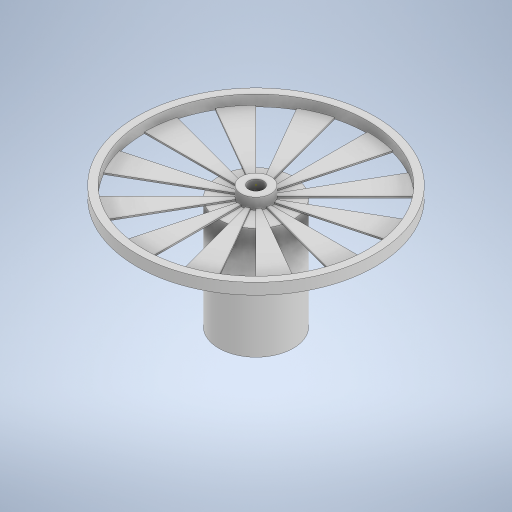
# Autodesk Inventor part: fan_num3
Saved by Autodesk Inventor 2024 (Build 280153000, 153)
## iProperties
Created: 2024-08-06
Part Number: fan_num3
Material: 일반
Document SubType Name: Modeling
Designer: chlqj
Density: 1 g/cm^3
Appearance: 기본값
Author: chlqj
Autodesk Inventor part; units mm, degrees
ref_plane "YZ Plane" through (0, 0, 0) normal (1, 0, 0) x (0, 1, 0)
ref_plane "XZ Plane" through (0, 0, 0) normal (0, 1, 0) x (-1, 0, 0)
ref_plane "XY Plane" through (0, 0, 0) normal (0, 0, 1) x (1, 0, 0)
sketch "스케치1" plane through (0, 0, 0) normal (0, 1, 0) x (-1, 0, 0)
  circle A0 centre (0, 0) radius 5
  dimension "d0" = 10
  constraints: 1 centre point, 1 coincident
  measures "d0" diameter of A0
extrude "돌출1" add sketch "스케치1" along normal blind 15
sketch "스케치2" plane through (0, 15, 0) normal (0, 1, 0) x (1, 0, 0)
  circle A0 centre (0, 0) radius 15
  circle A1 centre (0, 0) radius 16
  dimension "d3" = 30
  dimension "d4" = 32
  constraints: 2 centre point, 2 coincident
  measures "d3" diameter of A0
  measures "d4" diameter of A1
extrude "돌출2" add sketch "스케치2" along normal blind 1.5
sketch "스케치3" plane through (0, 15, 0) normal (0, 1, 0) x (1, 0, 0)
  line L0 (0, 0) -> (15, 0)
  circle A0 centre (0, 0) radius 15 projected
  line L1 (0, 0) -> (14.4889, 3.8823)
  line L2 (0, 0) -> (15, 0) construction
  line L3 (0, 0) -> (12.9904, 7.5)
  line L4 (0, 0) -> (15, 0) construction
  line L5 (0, 0) -> (10.6066, 10.6066)
  line L6 (0, 0) -> (15, 0) construction
  line L7 (0, 0) -> (7.5, 12.9904)
  line L8 (0, 0) -> (15, 0) construction
  line L9 (0, 0) -> (3.8823, 14.4889)
  line L10 (0, 0) -> (15, 0) construction
  line L11 (0, 0) -> (0, 15)
  line L12 (0, 0) -> (-3.8823, 14.4889)
  line L13 (0, 0) -> (-7.5, 12.9904)
  line L14 (0, 0) -> (-10.6066, 10.6066)
  line L15 (0, 0) -> (-12.9904, 7.5)
  line L16 (0, 0) -> (-14.2878, 3.8284)
  line L17 (0, 0) -> (-12.9904, -7.5)
  line L18 (0, 0) -> (-7.5, -12.9904)
  line L19 (0, 0) -> (0, -15)
  line L20 (0, 0) -> (10.6066, -10.6066)
  line L21 (0, 0) -> (12.9904, -7.5)
  line L22 (0, 0) -> (14.4889, -3.8823)
  line L23 (0, 0) -> (-15, 0)
  line L24 (0, 0) -> (-14.4889, -3.8823)
  line L25 (0, 0) -> (0, 0)
  line L26 (0, 0) -> (-10.6066, -10.6066)
  line L27 (0, 0) -> (-3.8823, -14.4889)
  line L28 (0, 0) -> (7.5, -12.9904)
  line L29 (0, 0) -> (3.8823, -14.4889)
  line L30 (0, 0) -> (-14.4889, 3.8823)
  dimension "d12" = 15
  dimension "d13" = 15
  dimension "d14" = 15
  dimension "d15" = 15
  dimension "d16" = 15
  dimension "d17" = 15
  dimension "d18" = 15
  dimension "d19" = 15
  dimension "d21" = 15
  dimension "d22" = 15
  dimension "d23" = 15
  dimension "d24" = 15
  dimension "d25" = 15
  dimension "d26" = 15
  dimension "d27" = 15
  dimension "d28" = 15
  dimension "d29" = 15
  dimension "d30" = 15
  dimension "d31" = 15
  dimension "d32" = 15
  dimension "d33" = 15
  dimension "d34" = 15
  dimension "d35" = 15
  dimension "d36" = 15
  dimension "d7" = 15
  dimension "d8" = 30
  dimension "d9" = 45
  dimension "d10" = 60
  dimension "d11" = 75
  dimension "d20" = 15
  constraints: 14 horizontal, 9 end point, 84 other
extrude "돌출3" add sketch "스케치3" along normal blind 0.2 contours L3 A0 L1 | L7 A0 L5 | L11 A0 L9 | L13 A0 L12 | L15 A0 L14 | L23 A0 L30 L16 | L21 A0 L20 | L0 A0 L22 | L17 A0 L24 | L18 A0 L26 | L19 A0 L27 | L28 A0 L29
sketch "스케치4" plane through (0, 16.5, 0) normal (0, 1, 0) x (1, 0, 0)
  line L0 (0, 0) -> (10.6066, 10.6066) projected
  circle A0 centre (0, 0) radius 2
  line L1 (0, 0) -> (14.4889, 3.8823) projected
  circle A1 centre (0, 0) radius 1
  dimension "d39" = 4
  dimension "d40" = 2
  constraints: 2 centre point, 2 coincident
  measures "d39" diameter of A0
  measures "d40" diameter of A1
extrude "돌출4" add sketch "스케치4" against normal blind 2 contours A1 L1 A0 L0 | L0 A0 L1 A1
sketch "스케치5" plane through (0, 16.5, 0) normal (0, 1, 0) x (1, 0, 0)
  point P0 (0, 0)
